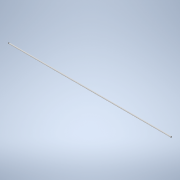
# Autodesk Inventor part: ropeeeeeexxx
Saved by Autodesk Inventor 2022 (Build 260153070, 153G)
## iProperties
Created: 2021-07-26
Part Number: ropeeeeeexxx
Material: Generic
Document SubType Name: Modeling
Designer: AKASH ARYAN
Density: 1 g/cm^3
Appearance: Default
Author: AKASH ARYAN
Autodesk Inventor part; units mm, degrees
ref_plane "YZ Plane" through (0, 0, 0) normal (1, 0, 0) x (0, 1, 0)
ref_plane "XZ Plane" through (0, 0, 0) normal (0, 1, 0) x (-1, 0, 0)
ref_plane "XY Plane" through (0, 0, 0) normal (0, 0, 1) x (1, 0, 0)
sketch "Sketch1" plane through (0, 0, 0) normal (1, 0, 0) x (0, 1, 0)
  circle A0 centre (0, 0) radius 10
  dimension "d0" = 20
  constraints: 1 centre point, 1 coincident
  measures "d0" diameter of A0
extrude "Extrusion1" add sketch "Sketch1" along normal blind 3000
body "Solid1"
